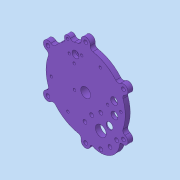
# Autodesk Inventor part: ThrustBearingMount
Saved by Autodesk Inventor 2017 (Build 210142000, 142)
## iProperties
Created: 2016-11-30
Part Number: ThrustBearingMount
Material: ABS Plastic
Document SubType Name: Modeling
Designer: techn
Density: 1.06 g/cm^3
Appearance: Violet
Mass: 29.2926 g
Surface Area: 151.195 cm^2
Volume: 27.6345 cm^3
Author: techn
Autodesk Inventor part; units mm, degrees
ref_plane "YZ Plane" through (0, 0, 0) normal (1, 0, 0) x (0, 1, 0)
ref_plane "XZ Plane" through (0, 0, 0) normal (0, 1, 0) x (-1, 0, 0)
ref_plane "XY Plane" through (0, 0, 0) normal (0, 0, 1) x (1, 0, 0)
sketch "Sketch5" plane through (0, 0, 0) normal (0, 0, 1) x (1, 0, 0)
  circle A0 centre (0, 0) radius 47.625
  dimension "d15" = 95.25
  constraints: 1 centre point, 1 coincident
  measures "d15" diameter of A0
extrude "Extrusion3" add sketch "Sketch5" along normal blind 4.7625
sketch "Sketch6" plane through (0, 0, 4.7625) normal (0, 0, 1) x (1, 0, 0)
  line L0 (0, 0) -> (0, 41.91)
  circle A0 centre (0, 41.91) radius 1.8415
  circle A1 centre (-36.2951, 20.955) radius 1.8415
  circle A2 centre (-36.2951, -20.955) radius 1.8415
  circle A3 centre (0, -41.91) radius 1.8415
  circle A4 centre (36.2951, -20.955) radius 1.8415
  circle A5 centre (36.2951, 20.955) radius 1.8415
  dimension "d18" = 41.91
  dimension "d19" = 3.683
  dimension "d22" = 360
  constraints: 6 centre point, 2 end point, 1 coincident, 1 vertical, 13 other
  measures "d18" distance of L0.start L0.end
  measures "d19" diameter of A0
extrude "Extrusion4" cut sketch "Sketch6" against normal blind 4.7625
sketch "Sketch7" plane through (0, 0, 0) normal (0, 0, -1) x (-1, 0, 0)
  circle A0 centre (0, 0) radius 12.192
  circle A1 centre (0, 0) radius 14.9225
  dimension "d26" = 24.384
  dimension "d27" = 29.845
  constraints: 2 centre point, 2 coincident
  measures "d26" diameter of A0
  measures "d27" diameter of A1
extrude "Extrusion5" add sketch "Sketch7" along normal blind 3.6068
sketch "Sketch9" plane through (0, 0, 0) normal (0, 0, -1) x (-1, 0, 0)
  circle A0 centre (0, 0) radius 4.7625
  dimension "d30" = 9.525
  constraints: 1 centre point, 1 coincident
  measures "d30" diameter of A0
extrude "Extrusion6" cut sketch "Sketch9" against normal through all
sketch "Sketch10" plane through (0, 0, 0) normal (0, 0, -1) x (-1, 0, 0)
  circle A0 centre (0, 0) radius 4.7625
  circle A1 centre (0, 0) radius 6.096
  dimension "d33" = 9.525
  dimension "d34" = 12.192
  constraints: 2 centre point, 2 coincident
  measures "d33" diameter of A0
  measures "d34" diameter of A1
extrude "Extrusion7" add sketch "Sketch10" along normal blind 3.6068
sketch "Sketch21" plane through (0, 0, 4.7625) normal (0, 0, 1) x (1, 0, 0)
  circle A0 centre (0, 0) radius 4.7625 projected
  line L0 (0, 0) -> (27.94, 0) construction
  circle A1 centre (23.0102, -16.2921) radius 3.302
  line L1 (23.0102, -16.2921) -> (14.5687, -24.7336)
  line L2 (23.0102, -16.2921) -> (34.9482, -16.2921) construction
  circle A2 centre (14.5687, -24.7336) radius 5.207
  circle A3 centre (14.5687, -24.7336) radius 18.034
  line L3 (14.5687, -24.7336) -> (14.5687, -9.4936)
  circle A4 centre (14.5687, -9.4936) radius 1.905
  circle A5 centre (-0.6713, -24.7336) radius 1.905
  circle A6 centre (14.5687, -39.9736) radius 1.905
  circle A7 centre (29.8087, -24.7336) radius 1.905
  line L4 (0, 0) -> (23.0102, -16.2921) construction
  dimension "d98" = 6.604
  dimension "d99" = 11.938
  dimension "d100" = 135
  dimension "d101" = 10.414
  dimension "d102" = 36.068
  dimension "d104" = 15.24
  dimension "d105" = 45
  dimension "d106" = 3.81
  dimension "d109" = 360
  dimension "d240" = 35.3
  dimension "d241" = 28.194
  constraints: 10 end point, 7 centre point, 3 coincident, 2 horizontal, 1 equal length, 9 other
  measures "d98" diameter of A1
  measures "d99" distance of L1.start L1.end
  measures "d100" angle of L1 L2
  measures "d101" diameter of A2
  measures "d102" diameter of A3
  measures "d104" distance of L3.start L3.end
  measures "d105" angle of L1 L3
  measures "d106" diameter of A4
  measures "d241" distance of L0.start L1.start
extrude "Extrusion19" cut sketch "Sketch21" against normal through all contours A1 | A2 L3 L1 | L1 L3 A2 | A4 | A5 | A6 | A7
sketch "Sketch22" plane through (0, 0, 0) normal (0, 0, -1) x (-1, 0, 0)
  circle A0 centre (-23.0102, -16.2921) radius 3.302 projected
  circle A1 centre (-23.0102, -16.2921) radius 8.4455
  point P0 (0, 0)
  dimension "d113" = 16.891
  constraints: 1 centre point, 1 coincident
  measures "d113" diameter of A1
extrude "Extrusion20" cut sketch "Sketch22" against normal blind 3.81
sketch "Sketch23" plane through (0, 0, 4.7625) normal (0, 0, 1) x (1, 0, 0)
  circle A0 centre (14.5687, -24.7336) radius 5.207 projected
  line L0 (14.5687, -24.7336) -> (5.7299, -15.8947)
  line L1 (14.5687, -24.7336) -> (27.0687, -24.7336) construction
  line L2 (14.5687, -24.7336) -> (23.4076, -33.5724)
  circle A1 centre (5.7299, -15.8947) radius 1.905
  circle A2 centre (23.4076, -33.5724) radius 1.905
  point P0 (0, 0)
  dimension "d116" = 12.5
  dimension "d117" = 135
  dimension "d118" = 3.81
  dimension "d119" = 3.81
  constraints: 6 end point, 2 centre point, 2 coincident, 2 equal length, 1 collinear, 1 horizontal
  measures "d116" distance of L0.start L0.end
  measures "d117" angle of L1 L0
  measures "d118" diameter of A1
  measures "d119" diameter of A2
extrude "Extrusion21" cut sketch "Sketch23" against normal through all contours A1 | A2
sketch "Sketch24" plane through (0, 0, 4.7625) normal (0, 0, 1) x (1, 0, 0)
  circle A0 centre (0, 0) radius 4.7625 projected
  line L0 (0, 0) -> (-9.7732, 26.8517)
  line L1 (0, 0) -> (28.575, 0) construction
  circle A1 centre (-9.7732, 26.8517) radius 3.3655
  circle A2 centre (-9.7732, 26.8517) radius 1.905
  line L2 (-9.7732, 26.8517) -> (-3.8062, 29.0235)
  line L3 (-9.7732, 26.8517) -> (-15.7403, 24.6799)
  circle A3 centre (-3.8062, 29.0235) radius 1.27
  circle A4 centre (-15.7403, 24.6799) radius 1.27
  dimension "d122" = 28.575
  dimension "d123" = 110
  dimension "d124" = 6.731
  dimension "d125" = 3.81
  dimension "d132" = 6.35
  dimension "d133" = 2.54
  dimension "d134" = 2.54
  constraints: 8 end point, 4 centre point, 4 coincident, 1 equal length, 1 horizontal, 1 perpendicular, 1 symmetric about line
  measures "d122" distance of L0.start L0.end
  measures "d123" angle of L1 L0
  measures "d124" diameter of A1
  measures "d125" diameter of A2
  measures "d132" distance of L2.start L2.end
  measures "d133" diameter of A3
  measures "d134" diameter of A4
extrude "Extrusion23" cut sketch "Sketch24" against normal blind 25.4 contours A2 L3 L0 | L0 L2 A2 | L3 A2 L2
extrude "Extrusion24" cut sketch "Sketch24" against normal blind 3.175 contours A1 L3 A2 L0 | L0 A2 L2 A1 | A1 L2 A2 L3
extrude "Extrusion25" cut sketch "Sketch24" against normal through all contours A3 | A4
sketch "Sketch26" plane through (0, 0, 4.7625) normal (0, 0, 1) x (1, 0, 0)
  circle A0 centre (-3.8062, 29.0235) radius 1.27 projected
  circle A1 centre (-9.7732, 26.8517) radius 3.3655 projected
  line L0 (-3.8062, 29.0235) -> (-9.7732, 26.8517)
  line L1 (-9.7732, 26.8517) -> (-13.6174, 37.4134)
  line L2 (-9.7732, 26.8517) -> (-7.3191, 20.109)
  line L3 (-13.6174, 37.4134) -> (-17.3169, 36.0669)
  line L4 (-13.6174, 37.4134) -> (7.7447, 45.1885)
  line L5 (-7.3191, 20.109) -> (-11.0186, 18.7624)
  line L6 (-7.3191, 20.109) -> (14.043, 27.8841)
  circle A2 centre (-17.3169, 36.0669) radius 1.27
  circle A3 centre (7.7447, 45.1885) radius 1.27
  circle A4 centre (14.043, 27.8841) radius 1.27
  circle A5 centre (-11.0186, 18.7624) radius 1.27
  point P0 (0, 0)
  dimension "d137" = 11.2395
  dimension "d139" = 3.937
  dimension "d140" = 22.733
  dimension "d142" = 2.54
  dimension "d143" = 2.54
  dimension "d144" = 2.54
  dimension "d145" = 2.54
  dimension "d148" = 7.1755
  constraints: 14 end point, 5 perpendicular, 4 centre point, 4 coincident, 2 parallel, 1 collinear
  measures "d137" distance of L0.end L1.end
  measures "d139" distance of L1.end L3.end
  measures "d140" distance of L1.end L4.end
  measures "d142" diameter of A2
  measures "d143" diameter of A3
  measures "d144" diameter of A4
  measures "d145" diameter of A5
  measures "d148" distance of L0.end L2.end
extrude "Extrusion27" cut sketch "Sketch26" against normal through all contours A2 | A4 | A5
sketch "Sketch28" plane through (0, 0, 4.7625) normal (0, 0, 1) x (1, 0, 0)
  circle A0 centre (-33.02, -3.175) radius 1.27
  circle A1 centre (-10.795, -3.175) radius 1.27
  point P0 (0, 0)
  dimension "d164" = 2.54
  dimension "d165" = 2.54
  dimension "d166" = 22.225
  dimension "d170" = 3.175
  dimension "d171" = 10.795
  constraints: 2 centre point, 1 horizontal alignment
  measures "d164" diameter of A0
  measures "d165" diameter of A1
  measures "d166" distance of A1.centre A0.centre
  measures "d170" vertical distance of point (0, 0) A1.centre
  measures "d171" horizontal distance of point (0, 0) A1.centre
extrude "Extrusion28" cut sketch "Sketch28" against normal up to surface (4.7625 mm away)
sketch "Sketch29" plane through (0, 0, 4.7625) normal (0, 0, 1) x (1, 0, 0)
  circle A0 centre (0, 0) radius 47.625 projected
  circle A1 centre (0, 0) radius 37.465
  line L0 (0, 0) -> (-43.1629, 20.1272)
  line L1 (0, 0) -> (47.625, 0) construction
  line L2 (0, 0) -> (-43.1629, -20.1272)
  line L3 (0, 0) -> (47.625, 0) construction
  line L4 (0, 0) -> (43.1629, 20.1272)
  line L5 (0, 0) -> (47.625, 0) construction
  line L6 (0, 0) -> (43.1629, -20.1272)
  line L7 (0, 0) -> (47.625, 0) construction
  arc A2 (-33.9548, 15.8334) -> (-33.9548, -15.8334) centre (0, 0) ccw
  arc A3 (33.9548, -15.8334) -> (33.9548, 15.8334) centre (0, 0) ccw
  line L8 (0, 0) -> (39.0121, 27.3166)
  line L9 (0, 0) -> (47.625, 0) construction
  line L10 (0, 0) -> (23.8125, 41.2445)
  line L11 (0, 0) -> (47.625, 0) construction
  arc A4 (39.0121, 27.3166) -> (23.8125, 41.2445) centre (0, 0) ccw
  arc A5 (30.6895, 21.489) -> (18.7325, 32.4456) centre (0, 0) ccw
  line L12 (0, 0) -> (-39.0121, 27.3166)
  line L13 (0, 0) -> (47.625, 0) construction
  line L14 (0, 0) -> (-23.8125, 41.2445)
  line L15 (0, 0) -> (47.625, 0) construction
  arc A6 (-23.8125, 41.2445) -> (-39.0121, 27.3166) centre (0, 0) ccw
  arc A7 (-18.7325, 32.4456) -> (-30.6895, 21.489) centre (0, 0) ccw
  circle A8 centre (-36.2951, 20.955) radius 1.8415 projected
  dimension "d172" = 10.16
  dimension "d173" = 155
  dimension "d174" = 155
  dimension "d175" = 25
  dimension "d176" = 25
  dimension "d179" = 35
  dimension "d180" = 60
  dimension "d181" = 145
  dimension "d182" = 120
  constraints: 32 end point, 20 point on circle, 8 equal length, 8 horizontal, 8 point on line, 6 centre point, 2 concentric, 13 other
  measures "d173" angle of L1 L0
  measures "d174" angle of L2 L3
  measures "d175" angle of L5 L4
  measures "d176" angle of L6 L7
  measures "d179" angle of L9 L8
  measures "d180" angle of L11 L10
  measures "d181" angle of L13 L12
  measures "d182" angle of L15 L14
sketch "Sketch31" plane through (0, 0, 4.7625) normal (0, 0, 1) x (1, 0, 0)
  circle A0 centre (-33.02, -3.175) radius 1.27 projected
  circle A1 centre (-10.795, -3.175) radius 1.27 projected
  circle A2 centre (14.043, 27.8841) radius 1.27 projected
  circle A3 centre (-17.3169, 36.0669) radius 1.27 projected
  circle A4 centre (-11.0186, 18.7624) radius 1.27 projected
  circle A5 centre (-3.8062, 29.0235) radius 1.27 projected
  circle A6 centre (-15.7403, 24.6799) radius 1.27 projected
  circle A7 centre (-9.7732, 26.8517) radius 3.3655 projected
  circle A8 centre (5.7299, -15.8947) radius 1.905 projected
  circle A9 centre (23.4076, -33.5724) radius 1.905 projected
  circle A10 centre (23.0102, -16.2921) radius 3.302 projected
  circle A11 centre (14.5687, -39.9736) radius 1.905 projected
  circle A12 centre (14.5687, -9.4936) radius 1.905 projected
  circle A13 centre (-0.6713, -24.7336) radius 1.905 projected
  circle A14 centre (29.8087, -24.7336) radius 1.905 projected
  circle A15 centre (14.5687, -24.7336) radius 5.207 projected
  circle A16 centre (0, 0) radius 4.7625 projected
  circle A17 centre (36.2951, -20.955) radius 1.8415 projected
  circle A18 centre (-36.2951, -20.955) radius 1.8415 projected
  circle A19 centre (0, 41.91) radius 1.8415 projected
  circle A20 centre (-36.2951, 20.955) radius 1.8415 projected
  circle A21 centre (0, -41.91) radius 1.8415 projected
  circle A22 centre (36.2951, 20.955) radius 1.8415 projected
  circle A23 centre (0, 0) radius 47.625 projected
  circle A24 centre (0, 41.91) radius 4.445
  circle A25 centre (-36.2951, 20.955) radius 4.445
  circle A26 centre (-36.2951, -20.955) radius 4.445
  circle A27 centre (0, -41.91) radius 4.445
  circle A28 centre (36.2951, -20.955) radius 4.445
  circle A29 centre (36.2951, 20.955) radius 4.445
  circle A30 centre (0, 0) radius 38.1
  circle A31 centre (-17.3169, 36.0669) radius 1.27 projected
  circle A32 centre (-17.3169, 36.0669) radius 3.175
  circle A33 centre (0, 0) radius 47.625 projected
  line L0 (0.0746, -47.6249) -> (0.0746, -38.0999)
  line L1 (0, 0) -> (41.2445, -23.8125)
  line L2 (0, 0) -> (47.625, 0) construction
  line L3 (41.2445, -23.8125) -> (32.9956, -19.05)
  dimension "d186" = 8.89
  dimension "d189" = 360
  dimension "d191" = 76.2
  dimension "d192" = 6.35
  dimension "d193" = 30
  constraints: 8 centre point, 8 end point, 4 point on circle, 3 coincident, 1 equal length, 1 horizontal, 1 point on line, 1 vertical, 15 other
  measures "d186" diameter of A24
  measures "d191" diameter of A30
  measures "d192" diameter of A32
  measures "d193" angle of L1 L2
extrude "Extrusion31" cut sketch "Sketch31" against normal blind 25.4 contours L1 A17 A30 A28 | A28 A30 A29 A24 A32 A25 A26 A27 L0 A23 L1 | A30 L0 A21 A27 | L1 A17 | A26 A30 | L0 A21 | A30 A29 | A25 A30 | A30 A24 | A32 A30 picked at (34.7909, -17.8998) picked at (-2.5577, -44.3748) picked at (36.2368, -20.3439) picked at (-32.9765, -20.5134) picked at (-0.5594, -41.8341) picked at (32.9765, 20.5134) picked at (-32.9765, 20.5134) picked at (-1.3186, 38.8417) picked at (-15.3506, 35.2677)
extrude "Extrusion32" add sketch "Sketch31" against normal up to surface (4.7625 mm away) contours A30 L1 A17 A28 | A28 L1 A30 | A30 A27 | A27 L0 A21 A30 | A28 A30 L1 | L1 A17 A30 A28 | A30 L0 A21 A27 | A30 A26 | A26 A30 | A30 A29 | A29 A30 | A30 A25 | A25 A30 | A30 A24 | A24 A30 | A32 A30 | A30 A32
sketch "Sketch32" plane through (0, 0, 4.7625) normal (0, 0, 1) x (1, 0, 0)
  arc A0 (34.0324, -17.129) -> (34.0324, 17.129) centre (0, 0) ccw projected
  arc A1 (34.0324, 17.129) -> (31.8504, 20.9085) centre (36.2951, 20.955) ccw projected
  arc A2 (31.8504, 20.9085) -> (2.1821, 38.0375) centre (0, 0) ccw projected
  arc A3 (2.1821, 38.0375) -> (-2.1821, 38.0375) centre (0, 41.91) ccw projected
  arc A4 (-2.1821, 38.0375) -> (-14.2251, 35.3448) centre (0, 0) ccw projected
  arc A5 (-14.2251, 35.3448) -> (-18.6868, 33.2026) centre (-17.3169, 36.0669) ccw projected
  arc A6 (-18.6868, 33.2026) -> (-31.8504, 20.9085) centre (0, 0) ccw projected
  arc A7 (-31.8504, 20.9085) -> (-34.0324, 17.129) centre (-36.2951, 20.955) ccw projected
  arc A8 (-34.0324, 17.129) -> (-34.0324, -17.129) centre (0, 0) ccw projected
  arc A9 (-34.0324, -17.129) -> (-31.8504, -20.9085) centre (-36.2951, -20.955) ccw projected
  arc A10 (-31.8504, -20.9085) -> (-2.1821, -38.0375) centre (0, 0) ccw projected
  arc A11 (-2.1821, -38.0375) -> (0.0746, -46.3544) centre (0, -41.91) ccw projected
  line L0 (0.0746, -46.3544) -> (0.0746, -47.6249) projected
  arc A12 (0.0746, -47.6249) -> (41.2445, -23.8125) centre (0, 0) ccw projected
  line L1 (41.2445, -23.8125) -> (40.1446, -23.1775) projected
  arc A13 (40.1446, -23.1775) -> (34.0324, -17.129) centre (36.2951, -20.955) ccw projected
  circle A14 centre (36.2951, 20.955) radius 1.8415 projected
  circle A15 centre (0, -41.91) radius 1.8415 projected
  circle A16 centre (-36.2951, 20.955) radius 1.8415 projected
  circle A17 centre (-17.3169, 36.0669) radius 1.27 projected
  circle A18 centre (0, 41.91) radius 1.8415 projected
  circle A19 centre (-36.2951, -20.955) radius 1.8415 projected
  circle A20 centre (36.2951, -20.955) radius 1.8415 projected
  circle A21 centre (-33.02, -3.175) radius 1.27 projected
  circle A22 centre (-10.795, -3.175) radius 1.27 projected
  circle A23 centre (14.043, 27.8841) radius 1.27 projected
  circle A24 centre (-11.0186, 18.7624) radius 1.27 projected
  circle A25 centre (-3.8062, 29.0235) radius 1.27 projected
  circle A26 centre (-15.7403, 24.6799) radius 1.27 projected
  circle A27 centre (-9.7732, 26.8517) radius 3.3655 projected
  circle A28 centre (5.7299, -15.8947) radius 1.905 projected
  circle A29 centre (23.4076, -33.5724) radius 1.905 projected
  circle A30 centre (23.0102, -16.2921) radius 3.302 projected
  circle A31 centre (14.5687, -39.9736) radius 1.905 projected
  circle A32 centre (14.5687, -9.4936) radius 1.905 projected
  circle A33 centre (-0.6713, -24.7336) radius 1.905 projected
  circle A34 centre (29.8087, -24.7336) radius 1.905 projected
  circle A35 centre (14.5687, -24.7336) radius 5.207 projected
  circle A36 centre (0, 0) radius 4.7625 projected
  circle A37 centre (14.5687, -24.7336) radius 18.415
  circle A38 centre (0, -41.91) radius 4.445
  circle A39 centre (36.2951, -20.955) radius 1.8415 projected
  circle A40 centre (36.2951, -20.955) radius 4.445
  arc A41 (3.8685, -39.7208) -> (32.9648, -23.899) centre (14.5687, -24.7336) ccw
  dimension "d198" = 36.83
  constraints: 8 point on circle, 4 centre point, 3 coincident, 1 concentric
  measures "d198" diameter of A37
extrude "Extrusion33" cut sketch "Sketch32" against normal blind 25.4 contours L1 A12 L0 A38 A37 A40
fillet "Fillet2" radius 1.5875 2 edges at (3.8685, -39.7208, 2.3813) (32.9648, -23.899, 2.3813)
fillet "Fillet3" radius 3.175 12 edges at (-2.1821, -38.0375, 2.3813) (-31.8504, -20.9085, 2.3813) (-34.0324, -17.129, 2.3813) (-34.0324, 17.129, 2.3813) (-31.8504, 20.9085, 2.3813) (-14.2251, 35.3448, 2.3813) (-18.6868, 33.2026, 2.3813) (2.1821, 38.0375, 2.3813) (-2.1821, 38.0375, 2.3813) (34.0324, 17.129, 2.3813) (31.8504, 20.9085, 2.3813) (34.0324, -17.129, 2.3813)
fillet "Fillet4" radius 0.635 2 edges at (15.226, -19.5682, 1.905) (19.7341, -24.0763, 1.905)
sketch "Sketch33" plane through (0, 0, 0) normal (0, 0, -1) x (-1, 0, 0)
  circle A0 centre (-23.0102, -16.2921) radius 3.302 projected
  circle A1 centre (-27.6896, -5.3094) radius 3.3655
  line L0 (0, 0) -> (-23.0102, -16.2921) construction
  line L1 (0, 0) -> (-27.6896, -5.3094) construction
  circle A2 centre (-27.4045, 6.6252) radius 3.3655
  line L2 (0, 0) -> (-27.4045, 6.6252) construction
  dimension "d204" = 6.731
  dimension "d205" = 11.938
  dimension "d209" = 11.938
  constraints: 6 end point, 2 centre point, 2 equal length, 1 equal radius
  measures "d204" diameter of A1
  measures "d205" distance of L1.end L0.end
  measures "d209" distance of L2.end L1.end
extrude "Extrusion34" cut sketch "Sketch33" against normal through all contours A1 | A2
sketch "Sketch34" plane through (0, 0, 0) normal (0, 0, -1) x (-1, 0, 0)
  circle A0 centre (-27.4045, 6.6252) radius 3.3655 projected
  arc A1 (-24.3241, -5.3094) -> (-24.3241, -5.3094) centre (-27.6896, -5.3094) ccw projected
  circle A2 centre (-27.4045, 6.6252) radius 5.08
  circle A3 centre (-27.6896, -5.3094) radius 5.08
  point P0 (0, 0)
  dimension "d210" = 10.16
  dimension "d211" = 10.16
  constraints: 2 centre point, 2 coincident
  measures "d210" diameter of A2
  measures "d211" diameter of A3
extrude "Extrusion35" cut sketch "Sketch34" against normal blind 1.5875 contours A0 | A1 | A2 | A3
sketch "Sketch35" plane through (0, 0, 0) normal (0, 0, -1) x (-1, 0, 0)
  circle A0 centre (-14.5687, -9.4936) radius 1.905 projected
  circle A1 centre (-5.7299, -15.8947) radius 1.905 projected
  circle A2 centre (-5.7299, -15.8947) radius 3.4925
  circle A3 centre (-14.5687, -9.4936) radius 3.4925
  point P0 (0, 0)
  dimension "d214" = 6.985
  dimension "d215" = 6.985
  constraints: 2 centre point, 2 coincident
  measures "d214" diameter of A2
  measures "d215" diameter of A3
extrude "Extrusion36" cut sketch "Sketch35" along normal through all
fillet "Fillet6" radius 1.27 4 edges at (2.4403, -14.7216, -1.8034) (7.5143, -12.8925, -1.8034) (11.1081, -9.9645, -1.8034) (13.6019, -6.1376, -1.8034)
sketch "Sketch36" plane through (0, 0, 0) normal (0, 0, -1) x (-1, 0, 0)
  circle A0 centre (-5.7299, -15.8947) radius 1.905 projected
  circle A1 centre (-23.4076, -33.5724) radius 1.905 projected
  circle A2 centre (-5.7299, -15.8947) radius 3.4925
  circle A3 centre (-23.4076, -33.5724) radius 3.4925
  point P0 (0, 0)
  dimension "d219" = 6.985
  dimension "d220" = 6.985
  constraints: 2 centre point, 2 coincident
  measures "d219" diameter of A2
  measures "d220" diameter of A3
extrude "Extrusion37" cut sketch "Sketch36" against normal blind 1.5875
sketch "Sketch37" plane through (0, 0, 4.7625) normal (0, 0, 1) x (1, 0, 0)
  circle A0 centre (27.4045, 6.6252) radius 3.3655 projected
  circle A1 centre (27.6896, -5.3094) radius 3.3655 projected
  circle A2 centre (33.8952, 0.8095) radius 1.27
  circle A3 centre (21.1989, 0.5063) radius 1.27
  line L0 (0, 0) -> (35.3791, 0.8449) construction
  line L1 (27.4045, 6.6252) -> (33.8952, 0.8095) construction
  arc A4 (28.9031, -10.2424) -> (23.2912, -7.8513) centre (27.6896, -5.3094) ccw construction
  line L2 (27.6896, -5.3094) -> (33.8952, 0.8095) construction
  line L3 (27.4045, 6.6252) -> (21.1989, 0.5063) construction
  line L4 (27.6896, -5.3094) -> (21.1989, 0.5063) construction
  dimension "d223" = 2.54
  dimension "d224" = 2.54
  dimension "d225" = 12.7
  constraints: 10 end point, 2 centre point, 2 equal length, 2 point on line
  measures "d223" diameter of A2
  measures "d224" diameter of A3
  measures "d225" distance of L3.end L1.end
extrude "Extrusion38" cut sketch "Sketch37" against normal through all contours A2 | A3
sketch "Sketch38" plane through (0, 0, 0) normal (0, 0, -1) x (-1, 0, 0)
  circle A0 centre (17.1184, -24.4476) radius 3.81
  circle A1 centre (17.1184, -24.4476) radius 1.27
  line L0 (0, 0) -> (17.1184, -24.4476) construction
  line L1 (0, 0) -> (29.845, 0) construction
  dimension "d228" = 29.845
  dimension "d229" = 55
  dimension "d230" = 7.62
  dimension "d231" = 2.54
  constraints: 4 end point, 2 centre point, 2 coincident, 1 equal length, 1 horizontal
  measures "d228" distance of L0.start L0.end
  measures "d229" angle of L0 L1
  measures "d230" diameter of A0
  measures "d231" diameter of A1
extrude "Extrusion39" add sketch "Sketch38" along normal blind 3.175
extrude "Extrusion40" cut sketch "Sketch38" against normal through all contours A1
fillet "Fillet7" radius 1.27 1 edges at (-13.3084, -24.4476, 0)
fillet "Fillet8" radius 1.27 2 edges at (23.2912, -7.8513, 0.7937) (28.9031, -10.2424, 0.7937)
body "Solid2"
